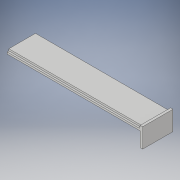
# Autodesk Inventor part: LampeSolaire2_Casing_Cover
Saved by Autodesk Inventor 2019 (Build 230136000, 136)
## iProperties
Created: 2020-09-25
Part Number: LampeSolaire2_Casing_Cover
Material: Generic
Document SubType Name: Modeling
Designer: nicolas
Density: 1 g/cm^3
Appearance: Default
Author: nicolas
Autodesk Inventor part; units mm, degrees
ref_plane "YZ Plane" through (0, 0, 0) normal (1, 0, 0) x (0, 1, 0)
ref_plane "XZ Plane" through (0, 0, 0) normal (0, 1, 0) x (-1, 0, 0)
ref_plane "XY Plane" through (0, 0, 0) normal (0, 0, 1) x (1, 0, 0)
sketch "Sketch2" plane through (0, 0, 0) normal (0, 1, 0) x (-1, 0, 0)
  line L0 (56, 11) -> (-56, 11)
  line L1 (-56, 11) -> (-56, -11)
  line L2 (-56, -11) -> (56, -11)
  line L3 (56, -11) -> (56, 11)
  line L4 (56, 11) -> (-56, -11) construction
  line L5 (-56, 11) -> (56, -11) construction
  point P0 (0, 0)
  dimension "d2" = 112
  dimension "d3" = 22
  constraints: 12 end point, 2 midpoint, 2 parallel, 1 horizontal, 1 perpendicular
  measures "d2" distance of L2.end L1.end
  measures "d3" distance of L1.end L0.end
extrude "Extrusion1" add sketch "Sketch2" along normal blind 3
sketch "Sketch4" plane through (-56, 0, 11) normal (0, 0, 1) x (1, 0, 0)
  line L0 (0, 0) -> (112, 0) projected
  line L1 (112, 0) -> (112, 3) projected
  line L2 (0, 0) -> (110, 0)
  line L3 (112, 0) -> (112, 1.5) construction
  line L4 (112, 1.5) -> (109.25, 1.5) construction
  line L5 (0, 1.5) -> (0, 0)
  line L6 (109.25, 1.5) -> (0, 1.5)
  line L7 (110, 0) -> (112, 0) construction
  line L8 (109.25, 1.5) -> (109.25, 3)
  line L9 (0, 3) -> (112, 3) projected
  line L10 (109.25, 3) -> (112, 3)
  line L11 (112, 3) -> (112, 0)
  line L12 (110, 0) -> (112, 0)
  point P0 (56, 0)
  dimension "d6" = 1.5
  dimension "d12" = 2.75
  constraints: 20 end point, 5 parallel, 3 perpendicular, 2 collinear, 2 horizontal, 1 midpoint, 1 vertical
  measures "d6" distance of L3.end L3.start
  measures "d12" distance of L8.end L1.end
extrude "Extrusion2" add sketch "Sketch4" along normal blind 1.5
mirror "Mirror1" about plane through (0, 0, 0) normal (0, 0, 1) of "Extrusion2"
sketch "Sketch6" plane through (0, 0, 0) normal (0, -1, 0) x (1, 0, 0)
  line L0 (56, 12.5) -> (53.25, 12.5) projected
  line L1 (-56, -12.5) -> (56, -12.5) projected
  line L2 (56, 12.5) -> (54, 12.5)
  line L3 (54, 12.5) -> (54, -12.5)
  line L4 (54, -12.5) -> (56, -12.5)
  line L5 (56, -12.5) -> (56, 12.5)
  point P0 (0, 0)
  dimension "d13" = 2
  constraints: 8 end point, 2 parallel, 1 horizontal, 1 perpendicular, 1 point on line
  measures "d13" distance of L4.end L3.end
extrude "Extrusion4" add sketch "Sketch6" along normal blind 12 and the other way blind 4
body "Solid1"
